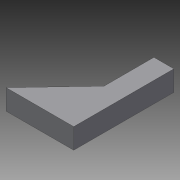
# Autodesk Inventor part: test_part
Saved by Autodesk Inventor 2015 SP1 (Build 190203100, 203)
## iProperties
Created: 2015-03-08
Part Number: test_part
Material: Generic
Document SubType Name: Modeling
Designer: Drew
Density: 1 g/cm^3
Appearance: Default
Author: Drew
Autodesk Inventor part; units mm, degrees
ref_plane "YZ Plane" through (0, 0, 0) normal (1, 0, 0) x (0, 1, 0)
ref_plane "XZ Plane" through (0, 0, 0) normal (0, 1, 0) x (-1, 0, 0)
ref_plane "XY Plane" through (0, 0, 0) normal (0, 0, 1) x (1, 0, 0)
sketch "Sketch1" plane through (0, 0, 0) normal (0, 1, 0) x (-1, 0, 0)
  line L0 (0, 0) -> (8.4217, 0)
  line L1 (8.4217, 0) -> (2.4841, -6.2608)
  line L2 (2.4841, -6.2608) -> (2.4841, -12.4812)
  line L3 (2.4841, -12.4812) -> (0, -12.4812)
  line L4 (0, -12.4812) -> (0, 0)
  constraints: 10 end point, 3 perpendicular, 1 horizontal
extrude "Extrusion1" add sketch "Sketch1" along normal blind 2.54
body "Solid1"
